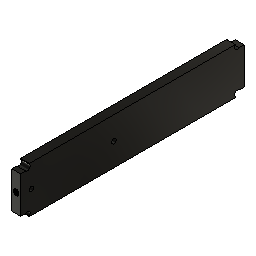
CameraHolder v2 (Autodesk Fusion 360 design; units mm, degrees)
Autodesk Fusion 360 part; units mm, degrees
sketch "Sketch1" plane through (0, 0, 0) normal (1, 0, 0) x (0, 1, 0)
  line L0 (-56, 10) -> (56, 10) construction
  line L1 (56, 10) -> (56, -10) construction
  line L2 (56, -10) -> (-56, -10) construction
  line L3 (-56, -10) -> (-56, 10) construction
  line L4 (-56, 10) -> (56, -10) construction
  line L5 (-60.8, 12.5) -> (60.8, 12.5) construction
  line L6 (60.8, 12.5) -> (60.8, -12.5) construction
  line L7 (60.8, -12.5) -> (-60.8, -12.5) construction
  line L8 (-60.8, -12.5) -> (-60.8, 12.5) construction
  line L9 (-60.8, 12.5) -> (60.8, -12.5) construction
  line L10 (-56, 10) -> (-57.0607, 11.0607) construction
  line L11 (-56, -10) -> (-57.0607, -11.0607) construction
  line L12 (56, 10) -> (57.0607, 11.0607) construction
  line L13 (56, -10) -> (57.0607, -11.0607) construction
  line L14 (56, 10) -> (60.8, 10) construction
  line L15 (56, 10) -> (56, 12.5) construction
  line L16 (56, -10) -> (60.8, -10) construction
  line L17 (56, -10) -> (56, -12.5) construction
  line L18 (-56, 10) -> (-60.8, 10) construction
  line L19 (-56, 10) -> (-56, 12.5) construction
  line L20 (-56, -10) -> (-60.8, -10) construction
  line L21 (-56, -10) -> (-56, -12.5) construction
  arc A0 (-58.1213, -10) -> (-56, -12.1213) centre (-57.0607, -11.0607) ccw construction
  arc A1 (-56, -10) -> (-58.1213, -10) centre (-57.0607, -11.0607) ccw
  arc A2 (-56, -12.1213) -> (-56, -10) centre (-57.0607, -11.0607) ccw
  arc A3 (-56, 12.1213) -> (-58.1213, 10) centre (-57.0607, 11.0607) ccw construction
  arc A4 (-58.1213, 10) -> (-56, 10) centre (-57.0607, 11.0607) ccw
  arc A5 (-56, 10) -> (-55.6075, 11.4325) centre (-57.0607, 11.0607) ccw
  arc A6 (-55.6075, 11.4325) -> (-56, 12.1213) centre (-57.0607, 11.0607) ccw
  arc A7 (58.1213, 10) -> (56, 12.1213) centre (57.0607, 11.0607) ccw construction
  arc A8 (56, 12.1213) -> (56, 10) centre (57.0607, 11.0607) ccw
  arc A9 (56, 10) -> (58.1213, 10) centre (57.0607, 11.0607) ccw
  arc A10 (56, -12.1213) -> (58.1213, -10) centre (57.0607, -11.0607) ccw construction
  arc A11 (58.1213, -10) -> (56, -10) centre (57.0607, -11.0607) ccw
  arc A12 (56, -10) -> (55.6075, -11.4325) centre (57.0607, -11.0607) ccw
  arc A13 (55.6075, -11.4325) -> (56, -12.1213) centre (57.0607, -11.0607) ccw
  line L22 (-58.1213, -10) -> (-60.8, -10)
  line L23 (-60.8, -10) -> (-60.8, 10)
  line L24 (-60.8, 10) -> (-58.1213, 10)
  line L25 (58.1213, -10) -> (60.8, -10)
  line L26 (60.8, -10) -> (60.8, 10)
  line L27 (60.8, 10) -> (58.1213, 10)
  line L28 (56, 12.1213) -> (56, 12.5)
  line L29 (56, 12.5) -> (-56, 12.5)
  line L30 (-56, 12.5) -> (-56, 12.1213)
  line L31 (-56, -12.1213) -> (-56, -12.5)
  line L32 (56, -12.5) -> (56, -12.1213)
  line L33 (56, -12.5) -> (-56, -12.5)
  line L34 (0, 0) -> (-60.8, 0) construction
  circle A14 centre (0, 0) radius 4 construction
  circle A15 centre (-10, 0) radius 1.25
  circle A16 centre (-55, 0) radius 1.25
  dimension "d1" = 112
  dimension "d2" = 20
  dimension "d3" = 121.6
  dimension "d4" = 25
  dimension "d5" = 1.5
  dimension "d6" = 135
  dimension "d7" = 1.5
  dimension "d8" = 135
  dimension "d9" = 1.5
  dimension "d10" = 1.5
  dimension "d11" = 135
  dimension "d13" = 135
  dimension "d14" = 8
  dimension "d15" = 2.5
  dimension "d16" = 2.5
  dimension "d17" = 45
  dimension "d18" = 10
  constraint horizontal L0
  constraint vertical L1
  constraint horizontal L2
  constraint vertical L3
  constraint midpoint L4 L34.start
  constraint coincident L34.start A14.centre
  constraint horizontal L5
  constraint vertical L6
  constraint horizontal L7
  constraint vertical L8
  constraint midpoint L9 L34.start
  constraint coincident L10.end A3.centre
  constraint coincident L11.end A0.centre
  constraint coincident L13.end A10.centre
  constraint coincident L12.end A7.centre
  constraint coincident L6 L14.end
  constraint perpendicular L6 L14
  constraint coincident L5 L15.end
  constraint perpendicular L5 L15
  constraint coincident L6 L16.end
  constraint perpendicular L6 L16
  constraint coincident L7 L17.end
  constraint perpendicular L7 L17
  constraint coincident L8 L18.end
  constraint perpendicular L8 L18
  constraint coincident L5 L19.end
  constraint perpendicular L5 L19
  constraint coincident L8 L20.end
  constraint perpendicular L8 L20
  constraint coincident L7 L21.end
  constraint perpendicular L7 L21
  constraint coincident L20 A0.start
  constraint concentric A0 A1
  constraint coincident L21 A0.end
  constraint concentric A0 A2
  constraint coincident L18 A3.end
  constraint concentric A3 A4
  constraint coincident L9 A5.end
  constraint concentric A3 A5
  constraint coincident L19 A3.start
  constraint concentric A3 A6
  constraint coincident L15 A7.end
  constraint concentric A7 A8
  constraint coincident L14 A7.start
  constraint concentric A7 A9
  constraint coincident L16 A10.end
  constraint concentric A10 A11
  constraint coincident L9 A12.end
  constraint concentric A10 A12
  constraint coincident L17 A10.start
  constraint concentric A10 A13
  constraint midpoint L23 L34.end
  constraint coincident L34 A15.centre
  constraint coincident L34 A16.centre
  measures "d1" distance of L0.start L0.end
  measures "d2" distance of L0.start L2.end
  measures "d3" distance of L5.start L5.end
  measures "d4" distance of L5.start L7.end
  measures "d5" distance of L0.start L10.end
  measures "d6" angle of L0 L10
  measures "d7" distance of L2.end L11.end
  measures "d8" angle of L2 L11
  measures "d9" distance of L0.end L12.end
  measures "d10" distance of L1.end L13.end
  measures "d11" angle of L0 L12
  measures "d13" angle of L2 L13
  measures "d14" diameter of A14
  measures "d15" diameter of A15
  measures "d16" diameter of A16
  measures "d17" distance of A15.centre A16.centre
  measures "d18" distance of L34.start A15.centre
extrude "Extrude1" add sketch "Sketch1" along normal blind 4.8
sketch "Sketch2" plane through (0, -60.8, 0) normal (0, -1, 0) x (1, 0, 0)
  line L0 (0, 10) -> (0, -10)
  line L1 (0, -10) -> (4.8, -10)
  line L2 (4.8, -10) -> (4.8, 10)
  line L3 (4.8, 10) -> (0, 10)
  line L4 (0, 10) -> (4.8, -10) construction
  circle A0 centre (2.4, 0) radius 1.5
  point P0 (2.4, 0)
  dimension "d21" = 3
  constraint coincident L0.start L3.end
  constraint coincident L1.end L2.start
  constraint midpoint L4 P0
  constraint coincident P0 A0.centre
  measures "d21" diameter of A0
sketch "Sketch3" plane through (0, 60.8, 0) normal (0, 1, 0) x (-1, 0, 0)
  line L0 (0, -10) -> (0, 10)
  line L1 (0, 10) -> (-4.8, 10)
  line L2 (-4.8, 10) -> (-4.8, -10)
  line L3 (-4.8, -10) -> (0, -10)
  line L4 (-4.8, 10) -> (0, -10) construction
  circle A0 centre (-2.4, 0) radius 1.5
  point P0 (-2.4, 0)
  dimension "d22" = 3
  constraint coincident L1.end L2.start
  constraint coincident L0.start L3.end
  constraint midpoint L4 P0
  constraint coincident P0 A0.centre
  measures "d22" diameter of A0
extrude "Extrude2" cut sketch "Sketch2" against normal blind 4 contours A0
extrude "Extrude3" cut sketch "Sketch3" against normal blind 8 contours A0
thread "Thread1" "ISO Metric profile 3.0 M3x0.5 6H" major diameter 3.086 minor diameter 2.529 pitch 0.5 angle 60 modelled right hand crest width 0.1368 on face at (3.8925, -59.4667, -0.1494) crest through (3.6645, -60.675, 0)
thread "Thread2" "ISO Metric profile 3.0 M3x0.5 6H" major diameter 3.086 minor diameter 2.529 pitch 0.5 angle 60 modelled right hand crest width 0.1368 on face at (0.9019, 55.4667, -0.0748) crest through (1.1355, 60.675, 0)
